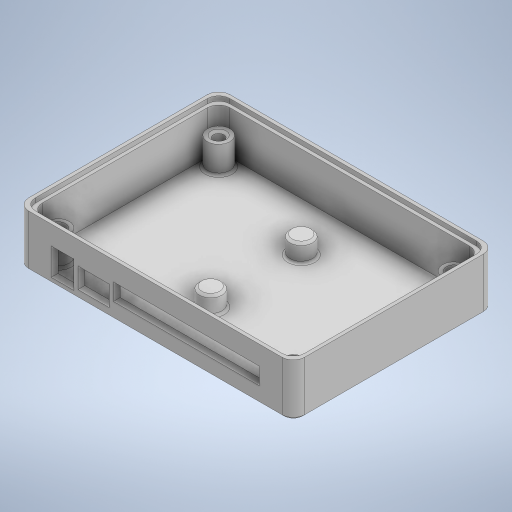
# Autodesk Inventor part: housing_base_v_2
Saved by Autodesk Inventor 2023 (Build 270158000, 158)
## iProperties
Created: 2023-10-04
Part Number: housing_base_v_2
Material: Generic
Document SubType Name: Modeling
Designer: mark
Density: 1 g/cm^3
Appearance: Default
Author: mark
Autodesk Inventor part; units mm, degrees
ref_plane "YZ Plane" through (0, 0, 0) normal (1, 0, 0) x (0, 1, 0)
ref_plane "XZ Plane" through (0, 0, 0) normal (0, 1, 0) x (-1, 0, 0)
ref_plane "XY Plane" through (0, 0, 0) normal (0, 0, 1) x (1, 0, 0)
sketch "Sketch1" plane through (0, 0, 0) normal (0, 1, 0) x (-1, 0, 0)
  line L0 (67.1673, -50.4691) -> (-54.8327, -50.4691)
  line L1 (-54.8327, -50.4691) -> (-54.8327, 38.5309)
  line L2 (-54.8327, 38.5309) -> (67.1673, 38.5309)
  line L3 (67.1673, 38.5309) -> (67.1673, -50.4691)
  point P0 (0, 0)
  dimension "d0" = 122
  dimension "d1" = 89
  constraints: 8 end point, 2 parallel, 1 horizontal, 1 perpendicular
  measures "d0" distance of L1.end L2.end
  measures "d1" distance of L0.end L1.end
extrude "Extrusion1" add sketch "Sketch1" along normal blind 2
sketch "Sketch2" plane through (0, 2, 0) normal (0, 1, 0) x (1, 0, 0)
  circle A0 centre (-58.1673, 41.4691) radius 2.35
  circle A1 centre (-58.1673, 41.4691) radius 5
  line L0 (-67.1673, 50.4691) -> (-67.1673, -38.5309) projected
  line L1 (54.8327, 50.4691) -> (-67.1673, 50.4691) projected
  point P0 (0, 0)
  dimension "d4" = 4.7
  dimension "d5" = 10
  dimension "d6" = 9
  dimension "d7" = 9
  constraints: 2 centre point, 1 coincident
  measures "d4" diameter of A0
  measures "d5" diameter of A1
  measures "d6" distance from line of L0 A0.centre
  measures "d7" distance from line of L1 A0.centre
extrude "Extrusion2" add sketch "Sketch2" along normal blind 12
fillet "Fillet1" radius 1 2 edges at (-63.1673, 2, -41.4691) (-60.5173, 2, -41.4691)
sketch "Sketch3" plane through (0, 2, 0) normal (0, 1, 0) x (1, 0, 0)
  line L0 (54.8327, 50.4691) -> (-67.1673, 50.4691) projected
  line L1 (-67.1673, -38.5309) -> (54.8327, -38.5309) projected
  line L2 (-67.1673, 50.4691) -> (54.8327, 50.4691)
  line L3 (54.8327, 50.4691) -> (54.8327, -38.5309)
  line L4 (54.8327, -38.5309) -> (-67.1673, -38.5309)
  line L5 (-67.1673, -38.5309) -> (-67.1673, 50.4691)
  line L6 (-64.1673, 47.4691) -> (51.8327, 47.4691)
  line L7 (51.8327, 47.4691) -> (51.8327, -35.5309)
  line L8 (51.8327, -35.5309) -> (-64.1673, -35.5309)
  line L9 (-64.1673, -35.5309) -> (-64.1673, 47.4691)
  point P0 (0, 0)
  point P1 (54.8327, 50.4691)
  point P2 (-67.1673, -38.5309)
  dimension "d11" = 3
  dimension "d12" = 3
  dimension "d13" = 3
  dimension "d14" = 3
  constraints: 16 end point, 4 parallel, 2 horizontal, 2 perpendicular
  measures "d11" distance between parallel lines of L6 L0
  measures "d12" distance between parallel lines of L5 L9
  measures "d13" distance between parallel lines of L1 L8
  measures "d14" distance between parallel lines of L3 L7
extrude "Extrusion3" add sketch "Sketch3" along normal blind 21
fillet "Fillet3" radius 5 8 edges at (54.8327, 11.5, 38.5309) (51.8327, 12.5, 35.5309) (-67.1673, 11.5, 38.5309) (-64.1673, 12.5, 35.5309) (-67.1673, 11.5, -50.4691) (-64.1673, 12.5, -47.4691) (54.8327, 11.5, -50.4691) (51.8327, 12.5, -47.4691)
chamfer "Chamfer2" distance 1 angle 45 8 edges at (-6.1673, 0, -50.4691) (-65.7028, 0, -49.0047) (-67.1673, 0, -5.9691) (-65.7028, 0, 37.0664) (-6.1673, 0, 38.5309) (53.3683, 0, 37.0664) (54.8327, 0, -5.9691) (53.3683, 0, -49.0047)
pattern_linear "Rectangular Pattern2" count 2 spacing 71 along (0, 0, 1) count 2 spacing 104 along (1, 0, 0) of "Extrusion2", "Fillet1"
sketch "Sketch5" plane through (0, 23, 0) normal (0, 1, 0) x (1, 0, 0)
  line L0 (-60.6673, 48.9691) -> (48.3327, 48.9691)
  line L1 (53.3327, 43.9691) -> (53.3327, -32.0309)
  line L2 (48.3327, -37.0309) -> (-60.6673, -37.0309)
  line L3 (-65.6673, -32.0309) -> (-65.6673, 43.9691)
  line L4 (54.8327, -33.5309) -> (54.8327, 45.4691) projected
  line L5 (-62.1673, -38.5309) -> (49.8327, -38.5309) projected
  line L6 (49.8327, 50.4691) -> (-62.1673, 50.4691) projected
  line L7 (-67.1673, 45.4691) -> (-67.1673, -33.5309) projected
  arc A0 (-60.6673, 48.9691) -> (-65.6673, 43.9691) centre (-60.6673, 43.9691) ccw
  arc A1 (53.3327, 43.9691) -> (48.3327, 48.9691) centre (48.3327, 43.9691) ccw
  arc A2 (48.3327, -37.0309) -> (53.3327, -32.0309) centre (48.3327, -32.0309) ccw
  arc A3 (-65.6673, -32.0309) -> (-60.6673, -37.0309) centre (-60.6673, -32.0309) ccw
  point P0 (0, 0)
  dimension "d37" = 1.5
  dimension "d38" = 1.5
  dimension "d39" = 1.5
  dimension "d40" = 1.5
  dimension "d41" = 5
  constraints: 8 end point, 8 point on circle, 8 tangent, 4 centre point, 3 equal radius, 2 parallel, 1 horizontal, 1 perpendicular
  measures "d37" distance between parallel lines of L4 L1
  measures "d38" distance between parallel lines of L5 L2
  measures "d39" distance between parallel lines of L6 L0
  measures "d40" distance between parallel lines of L7 L3
  measures "d41" radius of A0
extrude "Extrusion4" cut sketch "Sketch5" against normal blind 2
sketch "Sketch7" plane through (-62.1673, 23, 38.5309) normal (0, 0, 1) x (1, 0, 0)
  line L0 (10, -20.4) -> (37.5, -20.4)
  line L1 (102, -15.9) -> (102, -8.4)
  line L2 (10, -8.4) -> (10, -20.4)
  line L3 (-5, 0) -> (-5, -22) projected
  line L4 (0, -23) -> (112, -23) projected
  line L5 (37.5, -8.4) -> (37.5, -20.4)
  line L6 (37.5, -20.4) -> (20, -20.4)
  line L7 (20, -20.4) -> (20, -8.4)
  line L8 (37.5, -8.4) -> (102, -8.4)
  line L9 (102, -8.4) -> (102, -15.9)
  line L10 (102, -15.9) -> (37.5, -15.9)
  line L11 (37.5, -15.9) -> (37.5, -8.4)
  line L12 (21.85, -20.4) -> (35.65, -20.4)
  line L13 (102, -8.4) -> (37.5, -8.4)
  line L14 (21.85, -8.4) -> (10, -8.4)
  line L15 (35.65, -10.15) -> (21.85, -10.15)
  line L16 (21.85, -10.15) -> (21.85, -19.15)
  line L17 (21.85, -19.15) -> (35.65, -19.15)
  line L18 (35.65, -19.15) -> (35.65, -10.15)
  point P0 (62.1673, -23)
  point P1 (10, -14.4)
  point P2 (20, -14.4)
  point P3 (37.5, -15.9)
  point P4 (20, -20.4)
  point P5 (37.5, -8.4)
  dimension "d50" = 15
  dimension "d52" = 2.6
  dimension "d53" = 92
  dimension "d54" = 10
  dimension "d55" = 17.5
  dimension "d56" = 7.5
  dimension "d103" = 9
  dimension "d104" = 1.25
  dimension "d107" = 13.8
  constraints: 34 end point, 8 parallel, 4 horizontal, 3 perpendicular, 2 midpoint, 2 point on line
  measures "d50" distance from line of L3 point (10, -14.4)
  measures "d52" distance between parallel lines of L4 L0
  measures "d53" distance between parallel lines of L2 L1
  measures "d54" distance of point (10, -14.4) point (20, -14.4)
  measures "d55" distance between parallel lines of L7 L5
  measures "d56" distance of L1.start L8.end
  measures "d103" distance of L16.end L15.end
  measures "d104" distance between parallel lines of L17 L12
  measures "d107" distance of L15.start L15.end
extrude "Extrusion6" cut sketch "Sketch7" against normal blind 3
sketch "Sketch10" plane through (0, 2, 0) normal (0, 1, 0) x (1, 0, 0)
  line L0 (-67.1673, 45.4691) -> (-67.1673, -33.5309) projected
  line L1 (49.8327, 50.4691) -> (-62.1673, 50.4691) projected
  point P0 (0, 0)
  point P1 (-6.1673, 25.9691)
  dimension "d68" = 61
  dimension "d69" = 24.5
  measures "d68" distance from line of L0 point (-6.167, 25.969)
  measures "d69" distance from line of L1 point (-6.167, 25.969)
hole "Hole2" at (-6.1673, 2, -25.9691) direction (0, -1, 0) diameter 4.7 end through all
sketch "Sketch11" plane through (0, 2, 0) normal (0, 1, 0) x (1, 0, 0)
  line L0 (-67.1673, 45.4691) -> (-67.1673, -33.5309) projected
  line L1 (-62.1673, -38.5309) -> (49.8327, -38.5309) projected
  point P0 (0, 0)
  point P1 (-6.1673, -14.0309)
  dimension "d77" = 61
  dimension "d78" = 24.5
  measures "d77" distance from line of L0 point (-6.167, -14.031)
  measures "d78" distance from line of L1 point (-6.167, -14.031)
hole "Hole3" at (-6.1673, 2, 14.0309) direction (0, -1, 0) diameter 4.7 end through all
sketch "Sketch12" plane through (0, 2, 0) normal (0, 1, 0) x (1, 0, 0)
  circle A0 centre (-6.1673, 25.9691) radius 2.35 projected
  circle A1 centre (-6.1673, 25.9691) radius 2.35
  circle A2 centre (-6.1673, 25.9691) radius 5
  circle A3 centre (-6.1673, -14.0309) radius 2.35 projected
  circle A4 centre (-6.1673, -14.0309) radius 2.35
  circle A5 centre (-6.1673, -14.0309) radius 5
  point P0 (0, 0)
  dimension "d86" = 10
  dimension "d87" = 10
  dimension "d88" = 4.7
  constraints: 4 centre point, 4 coincident
  measures "d86" diameter of A2
  measures "d87" diameter of A5
  measures "d88" diameter of A4
extrude "Extrusion7" add sketch "Sketch12" along normal blind 7
sketch "Sketch13" plane through (-6.1673, 9, -25.9691) normal (0, 1, 0) x (1, 0, 0)
  circle A0 centre (0, 0) radius 2.35 projected
  circle A1 centre (0, 0) radius 5
  circle A2 centre (0, -40) radius 5 projected
  circle A3 centre (0, -40) radius 5
  point P0 (6.1673, -25.9691)
  constraints: 2 centre point, 2 coincident
extrude "Extrusion8" add sketch "Sketch13" along normal blind 1 contours A0 | A1 | A2
chamfer "Chamfer3" distance 1 angle 45 2 edges at (-11.1673, 10, -25.9691) (-11.1673, 10, 14.0309)
fillet "Fillet4" radius 1 2 edges at (-11.1673, 2, -25.9691) (-11.1673, 2, 14.0309)
chamfer "Chamfer4" distance 1 angle 45 6 edges at (-6.1673, 0, -28.3191) (-6.1673, 0, 11.6809) (43.4827, 14, -41.4691) (-60.5173, 14, -41.4691) (-60.5173, 14, 29.5309) (43.4827, 14, 29.5309)
equation "\"d12\" = d11"
equation "\"d13\" = d11"
equation "\"d14\" = d11"
equation "\"d38\" = d37"
equation "\"d39\" = d37"
equation "\"d40\" = d37"
body "Solid1"
